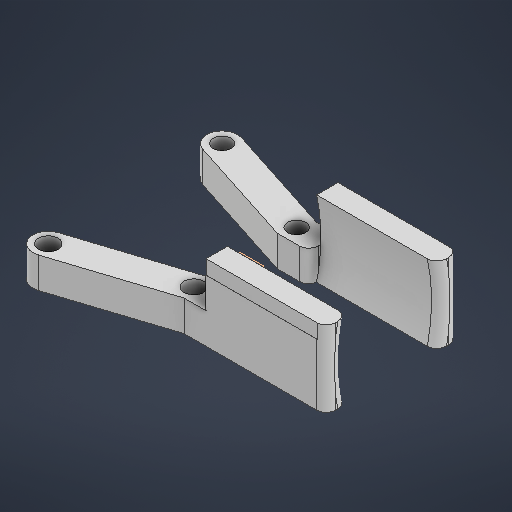
# Autodesk Inventor part: grips
Saved by Autodesk Inventor 2026.2 (Build 302298000, 298)
## iProperties
Created: 2026-04-07
Part Number: grips
Material: Generic
Document SubType Name: Modeling
Designer: Brian Wang
Density: 1 g/cm^3
Appearance: Default
Author: Brian Wang
Autodesk Inventor part; units mm, degrees
ref_plane "YZ Plane" through (0, 0, 0) normal (1, 0, 0) x (0, 1, 0)
ref_plane "XZ Plane" through (0, 0, 0) normal (0, 1, 0) x (-1, 0, 0)
ref_plane "XY Plane" through (0, 0, 0) normal (0, 0, 1) x (1, 0, 0)
sketch "Sketch1" plane through (0, 0, 0) normal (0, 1, 0) x (-1, 0, 0)
  line L0 (27.1998, -28.5532) -> (-70.2595, -28.5532)
  circle A0 centre (9.562, -47.3358) radius 2.075
  arc A1 (8.5638, -50.4287) -> (10.5601, -44.2429) centre (9.562, -47.3358) ccw
  circle A2 centre (-13.677, -39.8358) radius 2.075
  line L1 (10.5601, -44.2429) -> (-12.6789, -36.7429)
  line L2 (8.5638, -50.4287) -> (-14.6752, -42.9287)
  line L3 (-14.6752, -42.9287) -> (-44.6752, -42.9287)
  line L4 (-12.6789, -36.7429) -> (-19.3171, -36.7429)
  line L5 (-44.6752, -38.4058) -> (-44.6752, -42.9287)
  line L6 (-19.3171, -36.7429) -> (-44.6752, -38.4058)
  circle A3 centre (9.562, -9.7705) radius 2.075
  arc A4 (10.5601, -12.8635) -> (8.5638, -6.6776) centre (9.562, -9.7705) ccw
  circle A5 centre (-13.677, -17.2705) radius 2.075
  line L7 (10.5601, -12.8635) -> (-12.6789, -20.3635)
  line L8 (8.5638, -6.6776) -> (-14.6752, -14.1776)
  line L9 (-14.6752, -14.1776) -> (-44.6752, -14.1776)
  line L10 (-12.6789, -20.3635) -> (-19.3171, -20.3635)
  line L11 (-44.6752, -18.7005) -> (-44.6752, -14.1776)
  line L12 (-19.3171, -20.3635) -> (-44.6752, -18.7005)
  dimension "d26" = 4.15
  constraints: 26 end point, 10 symmetric about line, 6 centre point, 4 point on circle, 2 coincident, 1 horizontal, 3 other
  measures "d26" diameter of A2
extrude "Extrusion1" add sketch "Sketch1" along normal blind 3.5 contours L2 L3 L5 L6 L4 L1 A1
sketch "Sketch2" plane through (0, 3.5, 0) normal (0, 1, 0) x (1, 0, 0)
  line L0 (19.3171, 36.7429) -> (44.6752, 38.4058) projected
  line L1 (19.3171, 36.7429) -> (44.6752, 38.4058)
  line L2 (19.3171, 36.7429) -> (19.3171, 42.9287)
  line L3 (44.6752, 42.9287) -> (14.6752, 42.9287) projected
  line L4 (19.3171, 42.9287) -> (44.6752, 42.9287)
  line L5 (44.6752, 42.9287) -> (44.6752, 38.4058)
  point P0 (0, 0)
  point P1 (44.6752, 18.7005)
  point P2 (19.3171, 20.3635)
  point P3 (44.6752, 14.1776)
  constraints: 8 end point, 2 collinear, 1 perpendicular, 1 point on line, 1 vertical
extrude "Extrusion2" add sketch "Sketch2" along normal blind 6.5
sketch "Sketch4" plane through (0, 10, 0) normal (0, 1, 0) x (1, 0, 0)
  line L0 (19.3171, 36.7429) -> (44.6752, 38.4058) projected
  line L1 (19.3171, 36.7429) -> (19.3171, 42.9142)
  line L2 (19.3171, 42.9142) -> (44.6752, 42.9142)
  line L3 (44.6752, 38.4058) -> (44.6752, 42.9287) projected
  line L4 (44.6752, 42.9142) -> (44.6752, 38.4058)
  line L5 (44.6752, 38.4058) -> (19.3171, 36.7429)
  point P0 (0, 0)
  constraints: 8 end point, 1 collinear, 1 perpendicular, 1 vertical
extrude "Extrusion4" add sketch "Sketch4" along normal blind 3
sketch "Sketch5" plane through (0, 0, 0) normal (0, -1, 0) x (1, 0, 0)
  line L0 (14.6752, -42.9287) -> (-8.5638, -50.4287) projected
  line L1 (44.6752, -42.9287) -> (19.3171, -42.9287) projected
  line L2 (14.6752, -42.9287) -> (44.6752, -42.9287)
  line L3 (19.3171, -36.7429) -> (44.6752, -38.4058) projected
  line L4 (44.6752, -42.9287) -> (44.6752, -38.4058)
  line L5 (44.6752, -38.4058) -> (19.3171, -36.7429)
  line L6 (12.6789, -36.7429) -> (19.3171, -36.7429) projected
  line L7 (19.3171, -36.7429) -> (12.6789, -36.7429)
  line L8 (-10.5601, -44.2429) -> (12.6789, -36.7429) projected
  line L9 (12.6789, -36.7429) -> (-10.5601, -44.2429)
  arc A0 (-10.5601, -44.2429) -> (-8.5638, -50.4287) centre (-9.562, -47.3358) ccw
  circle A1 centre (-9.562, -47.3358) radius 1.9
  circle A2 centre (13.677, -39.8358) radius 1.9
  point P0 (0, 0)
  dimension "d27" = 3.8
  dimension "d28" = 3.8
  constraints: 10 end point, 3 centre point, 3 collinear, 2 coincident, 2 point on circle, 2 tangent, 1 parallel, 1 perpendicular
  measures "d27" diameter of A1
  measures "d28" diameter of A2
extrude "Extrusion5" add sketch "Sketch5" along normal blind 3
sketch "Sketch6" plane through (-9.562, 0, -47.3358) normal (0, 1, 0) x (1, 0, 0)
  circle A0 centre (0, 0) radius 1.9
  circle A1 centre (0, 0) radius 2.075
  circle A2 centre (23.239, -7.5) radius 1.9 projected
  circle A3 centre (23.239, -7.5) radius 1.9
  circle A4 centre (23.239, -7.5) radius 2.075
  point P0 (9.562, -47.3358)
  constraints: 4 centre point, 3 coincident
extrude "Extrusion6" add sketch "Sketch6" along normal up to surface (3.5 mm away)
sketch "Sketch7" plane through (44.6752, 10, -42.9142) normal (1, 0, 0) x (0, 0, -1)
  line L0 (-6.1713, 3) -> (-4.5084, 3) projected
  arc A0 (-4.5084, -13) -> (-4.5084, 3) centre (-40.1117, -5) ccw
  line L1 (0.0145, -13) -> (-4.5084, -13) projected
  line L2 (-4.5084, 3) -> (-14.8639, 3)
  line L3 (-14.8639, 3) -> (-14.8639, -13)
  line L4 (-14.8639, -13) -> (-4.5084, -13)
  line L5 (-4.5084, -13) -> (-4.5084, 3)
  point P0 (-42.9142, -10)
  constraints: 8 end point, 2 parallel, 2 point on circle, 1 centre point, 1 horizontal, 1 perpendicular
extrude "Extrusion7" cut sketch "Sketch7" against normal up to surface (25.3581 mm away)
fillet "Fillet4" radius 2 1 edges at (19.3171, 0.25, -36.7429)
fillet "Fillet5" radius 2 2 edges at (44.6752, 5, -39.2935) (44.6752, 3.5, -42.9287)
ref_plane "Work Plane1" through (12.6789, -3, -28.9929) normal (0, 0, 1) x (1, 0, 0)
mirror "Mirror1" about plane through (12.6789, -3, -28.9929) normal (0, 0, 1) of "Extrusion1", "Extrusion5", "Fillet4", "Extrusion7", "Extrusion4", "Fillet5", "Extrusion2"
body "Solid1"
